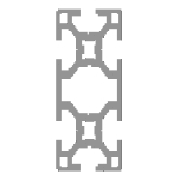
# Autodesk Inventor part: 30-3060
Saved by Autodesk Inventor 2021 (Build 250183000, 183)
## iProperties
Created: 2020-11-08
Part Number: 30-3060
Material: Generic
Document SubType Name: Modeling
Designer: Wes
Manufacturer: 8020
Standards Organization: 8020 Metric
Language: en-US
Size Designation: 30-3060
Categories: <MemberInstance><Categories><Category DisplayName="Structural Shapes" InternalName="089c4875-fa83-4c05-b084-43b9cc11f5ed" Mnemonic="GRDR"><CategoryParameter DisplayName="Mass per Length Unit" InternalName="0bb95a10-148f-4027-a459-38d7b056702a" Mnemonic="shpmass"/><CategoryParameter DisplayName="Section Area" InternalName="1ff91680-64b0-4202-b9a3-7fd3f94bba3b" Mnemonic="secarea"/><CategoryParameter DisplayName="Radius of Gyration (x)" InternalName="25778675-03e9-40c1-b6a8-4a9ed693320d" Mnemonic="gyrradx"/><CategoryParameter DisplayName="Torsional Rigidity Modulus" InternalName="26c1ec35-5026-4c63-ad0a-751cf684a536" Mnemonic="torrigmod"/><CategoryParameter DisplayName="Distance of the Center of Gravity X-X" InternalName="26c9bdb8-9c79-4b4f-a92e-8e197583c9c4" Mnemonic="grcendistX"/><CategoryParameter DisplayName="Legacy Member ID" InternalName="340afe4f-75d7-48d3-ab7d-943f3c3da468" Mnemonic="LegacyMemberID"/><CategoryParameter DisplayName="Base Length" InternalName="42e34263-8f20-4d0e-ad48-bf1385b87c24" Mnemonic="shplen"/><CategoryParameter DisplayName="Moment of Inertia (y)" InternalName="4b9f58ea-bced-460e-81ea-3d29ca5a49e3" Mnemonic="inermomy"/><CategoryParameter DisplayName="Moment of Inertia (x)" InternalName="4cd780bc-73d7-43ac-917a-579e5cbd684d" Mnemonic="inermomx"/><CategoryParameter DisplayName="Custom Base Point" InternalName="4f1d1b73-316d-484b-a3df-9cbabb16eb77" Mnemonic="shpBasePoint"/><CategoryParameter DisplayName="Shape Height" InternalName="50274e7d-5ac0-4796-92cb-c59e54983c67" Mnemonic="shpheig"/><CategoryParameter DisplayName="Section Module (y)" InternalName="59eaa5e9-d227-48dc-b6c1-6920f96e0f95" Mnemonic="secmody"/><CategoryParameter DisplayName="Section Designation" InternalName="5a64d034-428d-49c8-ba32-7619764de20f" Mnemonic="shpdes"/><CategoryParameter DisplayName="Section Module (x)" InternalName="72cfad18-cf51-4ed4-aaa7-c6b224f8419f" Mnemonic="secmodx"/><CategoryParameter DisplayName="Torsional Section Modulus" InternalName="7c55a8dc-8844-49f9-a867-cc677b30ec9a" Mnemonic="torsecmod"/><CategoryParameter DisplayName="Shape Width" InternalName="7c717d54-a18f-4666-b4d4-573cce22c62c" Mnemonic="shpwdth"/><CategoryParameter DisplayName="Second Shape Thickness" InternalName="9251a8e1-85fd-4e47-af99-afdb762317d9" Mnemonic="shpthick2"/><CategoryParameter DisplayName="FG Authored" InternalName="9c666724-f362-4ea7-ac62-f6a007de5c69" Mnemonic="shpFGAuto"/><CategoryParameter DisplayName="Distance of the Center of Gravity Y-Y" InternalName="bcc4fb17-7af4-436a-8f8c-d0aa3b0248c5" Mnemonic="grcendistY"/><CategoryParameter DisplayName="Radius of Gyration (y)" InternalName="bfa18ebe-1636-4dbe-8d42-b263e0b73184" Mnemonic="gyrrady"/><CategoryParameter DisplayName="Shape Thickness" InternalName="d109cf76-8eb4-42fc-9800-4409734adc67" Mnemonic="shpthick"/><CategoryParameter DisplayName="Coefficient of Shear Displacement" InternalName="de4c90c6-aaa8-468f-a335-6737b311b5d3" Mnemonic="shdispc"/><Category DisplayName="Other" InternalName="f02205ff-2390-476f-921c-0b3185f88e84" Mnemonic="OTHSHP"><CategoryParameter DisplayName="Moment of Inertia (y)" InternalName="044c654e-f649-48ac-84cc-650a29ae31ca" Mnemonic="inermomy"/><CategoryParameter DisplayName="Shape Thickness" InternalName="12b1a788-9233-48fd-a933-2df8ff42b15f" Mnemonic="shpthick"/><CategoryParameter DisplayName="Mass per Length Unit" InternalName="2fd289d6-9394-4d2d-97e6-6659d7d4551d" Mnemonic="shpmass"/><CategoryParameter DisplayName="Radius of Gyration (y)" InternalName="743e1dfe-1bba-408b-b985-cf752b207386" Mnemonic="gyrrady"/><CategoryParameter DisplayName="Section Module (y)" InternalName="88b8bff9-a616-4028-93d5-ed4f79680d13" Mnemonic="secmody"/><CategoryParameter DisplayName="Section Area" InternalName="c46ecdf8-b6eb-4db9-8b25-30258930c1e3" Mnemonic="secarea"/><CategoryParameter DisplayName="Section Module (x)" InternalName="cac70804-9d39-43bb-be17-56ea1f39a6c2" Mnemonic="secmodx"/><CategoryParameter DisplayName="Moment of Inertia (x)" InternalName="ec6737bc-264f-43ed-b0bd-f6d410c2718d" Mnemonic="inermomx"/><CategoryParameter DisplayName="Radius of Gyration (x)" InternalName="ee72c61e-565e-4fd6-b448-66e1e1abcb7e" Mnemonic="gyrradx"/><Category DisplayName="8020" InternalName="79851eee-1260-43d5-80eb-d25638456875" Mnemonic="8020"/></Category></Category><Category DisplayName="DataType" InternalName="23b78d0f-2648-40c6-8793-ca6db495c9e8" Mnemonic="DATATYPE"><CategoryParameter DisplayName="DisplayName" InternalName="05415f3d-3907-474b-a020-eb9d644f4cf3" Mnemonic="DISPLAYNAME"/><CategoryParameter DisplayName="Standard" InternalName="0c0a119c-1e12-4c84-803f-101930972f5e" Mnemonic="STANDARD"/><CategoryParameter DisplayName="Description" InternalName="13903e3d-64b1-4950-80da-f627842ea37f" Mnemonic="DESCRIPTION"/><CategoryParameter DisplayName="Designation" InternalName="2675968c-4ce5-49e0-a4f5-552d29089031" Mnemonic="DESIGNATION"/><CategoryParameter DisplayName="Default Row" InternalName="2af9ec52-faaa-4026-b378-f9fa4afca842" Mnemonic="DEFAULTROW"/><CategoryParameter DisplayName="Folder Name" InternalName="3f06958e-8713-4116-9be7-ed6184ecc97b" Mnemonic="FOLDERNAME"/><CategoryParameter DisplayName="Revision Guid" InternalName="45a75005-10b1-4dfc-8d6d-dfe629f0b93c" Mnemonic="REVISIONGUID"/><CategoryParameter DisplayName="FileName" InternalName="8b46a4cc-9585-4fed-90c3-899f57e09a73" Mnemonic="FILENAME"/><CategoryParameter DisplayName="StdsOrg" InternalName="8f5914e1-4693-403f-8ab5-d37768198c9d" Mnemonic="STDSORG"/><CategoryParameter DisplayName="Family Version" InternalName="914462f6-6e19-4b14-ba84-155b9680b1d0" Mnemonic="FAMILYREVISION"/><CategoryParameter DisplayName="Standard Revision" InternalName="91d5a463-65c2-4fde-b823-3b7fea5e8e17" Mnemonic="STANDARDREVISION"/><CategoryParameter DisplayName="Member Revision" InternalName="a65d44b9-392f-4f4f-857b-e4b3d54996fe" Mnemonic="MEMBERREVISION"/><CategoryParameter DisplayName="ClipFormat" InternalName="bc51e27b-3422-4e78-93ef-cec197ddf230" Mnemonic="CLIPFORMAT"/><CategoryParameter DisplayName="Manufacturer" InternalName="cd6c7a72-a28a-4e50-99a9-2c7f4e13e5ad" Mnemonic="MANUFACTURER"/><CategoryParameter DisplayName="InternalName" InternalName="cf1d0246-76d9-4b4a-8305-fa0409afb5c1" Mnemonic="INTERNALNAME"/><CategoryParameter DisplayName="IsMetric" InternalName="e2385c5b-1ea4-4823-96a8-8de651266ec3" Mnemonic="ISMETRIC"/><Category DisplayName="Part" InternalName="c0e0b642-3bcb-4cc8-9e80-f96d35c4afa4" Mnemonic="PART"><CategoryParameter DisplayName="Part Number" InternalName="016b6077-bfbe-49bd-92c9-d8d59c39c941" Mnemonic="PARTNUMBER"/><CategoryParameter DisplayName="Stock Number" InternalName="4dba7c1c-e26c-444e-836c-b08b433409a8" Mnemonic="STOCKNUMBER"/><CategoryParameter DisplayName="Material Key" InternalName="5c9a8adb-dd2b-4535-b97f-0a94a95fe41f" Mnemonic="MATERIALKEY"/><CategoryParameter DisplayName="Material" InternalName="818a152a-d3c3-49ca-80ee-df7d91421b8e" Mnemonic="MATERIAL"/></Category></Category></Categories><FamilyTemplate Id="30-3060"><FamilyTemplateParameters><FamilyTemplateParameter ObjectType="kModelParameterObject" ValueType="xs:double" Id="12" ObjectReferenceKey="Length"/><FamilyTemplateParameter ObjectType="kPartComponentDefinitionObject" ValueType="xs:string" Id="23" SubObjectId="Material"/><FamilyTemplateParameter ObjectType="kPropertyObject" ValueType="xs:string" Id="26" ObjectReferenceKey="{32853F0F-3444-11d1-9E93-0060B03C1CA6}" SubObjectId="5"/><FamilyTemplateParameter ObjectType="kPropertyObject" ValueType="xs:string" Id="27" ObjectReferenceKey="{32853F0F-3444-11d1-9E93-0060B03C1CA6}" SubObjectId="52"/></FamilyTemplateParameters></FamilyTemplate><CategoryParameterMap><ParamToTemplateMap><ParamToTemplate CategoryParameter="//CategoryParameter[@InternalName='cf1d0246-76d9-4b4a-8305-fa0409afb5c1']" ConstantValue="ebd6c703-6585-4f80-969f-cab21f52a046"/><ParamToTemplate CategoryParameter="//CategoryParameter[@InternalName='45a75005-10b1-4dfc-8d6d-dfe629f0b93c']" ConstantValue="7500c355-f6d2-45da-9c20-dd8006f12ffd"/><ParamToTemplate CategoryParameter="//CategoryParameter[@InternalName='3f06958e-8713-4116-9be7-ed6184ecc97b']" ConstantValue="30-3060"/><ParamToTemplate CategoryParameter="//CategoryParameter[@InternalName='8f5914e1-4693-403f-8ab5-d37768198c9d']" ConstantValue="8020 Metric"/><ParamToTemplate CategoryParameter="//CategoryParameter[@InternalName='0c0a119c-1e12-4c84-803f-101930972f5e']" TemplateParameter="18"/><ParamToTemplate CategoryParameter="//CategoryParameter[@InternalName='91d5a463-65c2-4fde-b823-3b7fea5e8e17']" TemplateParameter="19"/><ParamToTemplate CategoryParameter="//CategoryParameter[@InternalName='cd6c7a72-a28a-4e50-99a9-2c7f4e13e5ad']" ConstantValue="8020"/><ParamToTemplate CategoryParameter="//CategoryParameter[@InternalName='13903e3d-64b1-4950-80da-f627842ea37f']" TemplateParameter="22"/><ParamToTemplate CategoryParameter="//CategoryParameter[@InternalName='05415f3d-3907-474b-a020-eb9d644f4cf3']" ConstantValue="30-3060"/><ParamToTemplate CategoryParameter="//CategoryParameter[@InternalName='914462f6-6e19-4b14-ba84-155b9680b1d0']" ConstantValue="11"/><ParamToTemplate CategoryParameter="//CategoryParameter[@InternalName='bc51e27b-3422-4e78-93ef-cec197ddf230']" ConstantValue="CF_INVENTOR.STDPARTS"/><ParamToTemplate CategoryParameter="//CategoryParameter[@InternalName='e2385c5b-1ea4-4823-96a8-8de651266ec3']" ConstantValue="false"/><ParamToTemplate CategoryParameter="//CategoryParameter[@InternalName='2af9ec52-faaa-4026-b378-f9fa4afca842']" ConstantValue="1"/><ParamToTemplate CategoryParameter="//CategoryParameter[@InternalName='4f1d1b73-316d-484b-a3df-9cbabb16eb77']" ConstantValue="1"/><ParamToTemplate CategoryParameter="//CategoryParameter[@InternalName='9c666724-f362-4ea7-ac62-f6a007de5c69']" ConstantValue="1"/><ParamToTemplate CategoryParameter="//CategoryParameter[@InternalName='8b46a4cc-9585-4fed-90c3-899f57e09a73']" ConstantValue="30-3060"/><ParamToTemplate CategoryParameter="//CategoryParameter[@InternalName='a65d44b9-392f-4f4f-857b-e4b3d54996fe']" ConstantValue="3621f859-3cd7-4c8d-9d7e-184ee6a29b8c"/><ParamToTemplate CategoryParameter="//CategoryParameter[@InternalName='a65d44b9-392f-4f4f-857b-e4b3d54996fe']" ConstantValue="3621f859-3cd7-4c8d-9d7e-184ee6a29b8c"/><ParamToTemplate CategoryParameter="//CategoryParameter[@InternalName='2675968c-4ce5-49e0-a4f5-552d29089031']" TemplateParameter="27"/><ParamToTemplate CategoryParameter="//CategoryParameter[@InternalName='42e34263-8f20-4d0e-ad48-bf1385b87c24']" TemplateParameter="12"/><ParamToTemplate CategoryParameter="//CategoryParameter[@InternalName='818a152a-d3c3-49ca-80ee-df7d91421b8e']" TemplateParameter="23"/><ParamToTemplate CategoryParameter="//CategoryParameter[@InternalName='016b6077-bfbe-49bd-92c9-d8d59c39c941']" TemplateParameter="26"/></ParamToTemplateMap></CategoryParameterMap></MemberInstance>
Density: 1 g/cm^3
Appearance: Default
_CCFamilyDisplayName: 30-3060
_FrameMemberDoc: Frame Member File
_Version: 15.0.0
_GetPNFromCC: 1
IsCustomPart: 1
G_W: 1.181 in
G_H: 2.362 in
+1E485C6B-74E4-4670-9E51-72C930FDFDFE+CUTDETAIL2: Cut Angle 90.00 deg
G_L: 30.472 in
+ECDC0DF4-1E61-4BE6-A4E6-B4BFEEAFBB01+CUTDETAIL1: Cut Angle 90.00 deg
Author: Wes
Autodesk Inventor part; units mm, degrees
sketch "30-3060" plane through (0, 0, 0) normal (0, 0, 1) x (1, 0, 0)
  arc A0 (20.0319, 67.4331) -> (20.4119, 67.0531) centre (20.4119, 67.4331) ccw
  line L0 (20.4119, 67.0531) -> (23.8509, 67.0531)
  arc A1 (23.8509, 67.0531) -> (24.2319, 67.4341) centre (23.8509, 67.4341) ccw
  line L1 (24.2319, 67.4341) -> (24.2319, 70.2531)
  arc A2 (24.2319, 70.2531) -> (23.2319, 71.2531) centre (23.2319, 70.2531) ccw
  line L2 (23.2319, 71.2531) -> (20.4129, 71.2531)
  arc A3 (20.4129, 71.2531) -> (20.0319, 70.8721) centre (20.4129, 70.8721) ccw
  line L3 (20.0319, 70.8721) -> (20.0319, 67.4331)
  arc A4 (14.357, 59.8716) -> (12.8504, 61.3782) centre (13.5193, 60.5405) ccw
  line L4 (12.8504, 61.3782) -> (11.8713, 60.5964)
  arc A5 (11.8713, 60.5964) -> (9.1833, 60.5923) centre (10.5319, 57.5531) ccw
  line L5 (9.1833, 60.5923) -> (8.2041, 61.3741)
  arc A6 (8.2041, 61.3741) -> (6.6976, 59.8675) centre (7.5353, 60.5364) ccw
  line L6 (6.6976, 59.8675) -> (7.4842, 58.8824)
  arc A7 (7.4842, 58.8824) -> (7.4886, 56.2137) centre (10.5319, 57.5531) ccw
  line L7 (7.4886, 56.2137) -> (6.7068, 55.2346)
  arc A8 (6.7068, 55.2346) -> (8.2134, 53.728) centre (7.5445, 54.5657) ccw
  line L8 (8.2134, 53.728) -> (9.1925, 54.5098)
  arc A9 (9.1925, 54.5098) -> (11.8713, 54.5098) centre (10.5319, 57.5531) ccw
  line L9 (11.8713, 54.5098) -> (12.8504, 53.728)
  arc A10 (12.8504, 53.728) -> (14.357, 55.2346) centre (13.5193, 54.5657) ccw
  line L10 (14.357, 55.2346) -> (13.5752, 56.2137)
  arc A11 (13.5752, 56.2137) -> (13.5752, 58.8925) centre (10.5319, 57.5531) ccw
  line L11 (13.5752, 58.8925) -> (14.357, 59.8716)
  arc A12 (14.357, 29.8717) -> (12.8504, 31.3783) centre (13.5193, 30.5406) ccw
  line L12 (12.8504, 31.3783) -> (11.8713, 30.5965)
  arc A13 (11.8713, 30.5965) -> (9.1833, 30.5924) centre (10.5319, 27.5532) ccw
  line L13 (9.1833, 30.5924) -> (8.2041, 31.3742)
  arc A14 (8.2041, 31.3742) -> (6.6976, 29.8676) centre (7.5353, 30.5365) ccw
  line L14 (6.6976, 29.8676) -> (7.4842, 28.8824)
  arc A15 (7.4842, 28.8824) -> (7.4886, 26.2138) centre (10.5319, 27.5532) ccw
  line L15 (7.4886, 26.2138) -> (6.7068, 25.2347)
  arc A16 (6.7068, 25.2347) -> (8.2134, 23.7281) centre (7.5445, 24.5658) ccw
  line L16 (8.2134, 23.7281) -> (9.1925, 24.5099)
  arc A17 (9.1925, 24.5099) -> (11.8713, 24.5099) centre (10.5319, 27.5532) ccw
  line L17 (11.8713, 24.5099) -> (12.8504, 23.7281)
  arc A18 (12.8504, 23.7281) -> (14.357, 25.2347) centre (13.5193, 24.5658) ccw
  line L18 (14.357, 25.2347) -> (13.5752, 26.2138)
  arc A19 (13.5752, 26.2138) -> (13.5752, 28.8926) centre (10.5319, 27.5532) ccw
  line L19 (13.5752, 28.8926) -> (14.357, 29.8717)
  arc A20 (23.2319, 13.8532) -> (24.2319, 14.8532) centre (23.2319, 14.8532) ccw
  line L20 (24.2319, 14.8532) -> (24.2319, 17.6722)
  arc A21 (24.2319, 17.6722) -> (23.8509, 18.0532) centre (23.8509, 17.6722) ccw
  line L21 (23.8509, 18.0532) -> (20.4119, 18.0532)
  arc A22 (20.4119, 18.0532) -> (20.0319, 17.6732) centre (20.4119, 17.6732) ccw
  line L22 (20.0319, 17.6732) -> (20.0319, 14.2342)
  arc A23 (20.0319, 14.2342) -> (20.4129, 13.8532) centre (20.4129, 14.2342) ccw
  line L23 (20.4129, 13.8532) -> (23.2319, 13.8532)
  line L24 (-2.2106, 49.8206) -> (-2.2106, 52.9906)
  arc A24 (-2.2106, 49.8206) -> (-1.7109, 49.3031) centre (-1.7109, 49.8031) ccw
  line L25 (0.2717, 49.3031) -> (-1.7109, 49.3031)
  arc A25 (0.2717, 49.3031) -> (0.6252, 49.4496) centre (0.2717, 49.8031) ccw
  line L26 (4.5508, 53.3751) -> (0.6252, 49.4496)
  arc A26 (4.5508, 53.3751) -> (4.6972, 53.7287) centre (4.1972, 53.7287) ccw
  line L27 (4.6972, 56.6031) -> (4.6972, 53.7287)
  line L28 (5.2072, 57.5531) -> (4.6972, 56.6031)
  line L29 (4.6972, 58.5031) -> (5.2072, 57.5531)
  line L30 (4.6972, 61.3776) -> (4.6972, 58.5031)
  arc A27 (4.6972, 61.3776) -> (4.5508, 61.7311) centre (4.1972, 61.3776) ccw
  line L31 (0.6252, 65.6567) -> (4.5508, 61.7311)
  arc A28 (0.6252, 65.6567) -> (0.2717, 65.8031) centre (0.2717, 65.3031) ccw
  line L32 (-1.7109, 65.8031) -> (0.2717, 65.8031)
  arc A29 (-1.7109, 65.8031) -> (-2.2106, 65.2857) centre (-1.7109, 65.3031) ccw
  line L33 (-2.2106, 61.9906) -> (-2.2106, 65.2857)
  arc A30 (-2.7106, 61.4906) -> (-2.2106, 61.9906) centre (-2.7106, 61.9906) ccw
  line L34 (-3.9681, 61.4906) -> (-2.7106, 61.4906)
  arc A31 (-4.4681, 61.9906) -> (-3.9681, 61.4906) centre (-3.9681, 61.9906) ccw
  line L35 (-4.4681, 70.5531) -> (-4.4681, 61.9906)
  arc A32 (-2.4681, 72.5531) -> (-4.4681, 70.5531) centre (-2.4681, 70.5531) ccw
  line L36 (5.9694, 72.5531) -> (-2.4681, 72.5531)
  arc A33 (6.4694, 72.0531) -> (5.9694, 72.5531) centre (5.9694, 72.0531) ccw
  line L37 (6.4694, 70.7956) -> (6.4694, 72.0531)
  arc A34 (5.9694, 70.2956) -> (6.4694, 70.7956) centre (5.9694, 70.7956) ccw
  line L38 (2.7994, 70.2956) -> (5.9694, 70.2956)
  arc A35 (2.7994, 70.2956) -> (2.2819, 69.7959) centre (2.7819, 69.7959) ccw
  line L39 (2.2819, 67.8133) -> (2.2819, 69.7959)
  arc A36 (2.2819, 67.8133) -> (2.4284, 67.4598) centre (2.7819, 67.8133) ccw
  line L40 (6.3539, 63.5342) -> (2.4284, 67.4598)
  arc A37 (6.3539, 63.5342) -> (6.7074, 63.3878) centre (6.7074, 63.8878) ccw
  line L41 (9.5194, 63.3878) -> (6.7074, 63.3878)
  line L42 (10.4694, 62.8778) -> (9.5194, 63.3878)
  line L43 (11.4194, 63.3878) -> (10.4694, 62.8778)
  line L44 (14.3564, 63.3878) -> (11.4194, 63.3878)
  arc A38 (14.3564, 63.3878) -> (14.7099, 63.5342) centre (14.3564, 63.8878) ccw
  line L45 (18.6354, 67.4598) -> (14.7099, 63.5342)
  arc A39 (18.6354, 67.4598) -> (18.7819, 67.8133) centre (18.2819, 67.8133) ccw
  line L46 (18.7819, 69.7959) -> (18.7819, 67.8133)
  arc A40 (18.7819, 69.7959) -> (18.2644, 70.2956) centre (18.2819, 69.7959) ccw
  line L47 (14.9694, 70.2956) -> (18.2644, 70.2956)
  arc A41 (14.4694, 70.7956) -> (14.9694, 70.2956) centre (14.9694, 70.7956) ccw
  line L48 (14.4694, 72.0531) -> (14.4694, 70.7956)
  arc A42 (14.9694, 72.5531) -> (14.4694, 72.0531) centre (14.9694, 72.0531) ccw
  line L49 (23.5319, 72.5531) -> (14.9694, 72.5531)
  arc A43 (25.5319, 70.5531) -> (23.5319, 72.5531) centre (23.5319, 70.5531) ccw
  line L50 (25.5319, 62.1156) -> (25.5319, 70.5531)
  arc A44 (25.0319, 61.6156) -> (25.5319, 62.1156) centre (25.0319, 62.1156) ccw
  line L51 (23.7744, 61.6156) -> (25.0319, 61.6156)
  arc A45 (23.2744, 62.1156) -> (23.7744, 61.6156) centre (23.7744, 62.1156) ccw
  line L52 (23.2744, 65.2857) -> (23.2744, 62.1156)
  arc A46 (23.2744, 65.2857) -> (22.7747, 65.8031) centre (22.7747, 65.3031) ccw
  line L53 (20.7921, 65.8031) -> (22.7747, 65.8031)
  arc A47 (20.7921, 65.8031) -> (20.4386, 65.6567) centre (20.7921, 65.3031) ccw
  line L54 (16.513, 61.7311) -> (20.4386, 65.6567)
  arc A48 (16.513, 61.7311) -> (16.3666, 61.3776) centre (16.8666, 61.3776) ccw
  line L55 (16.3666, 58.5031) -> (16.3666, 61.3776)
  line L56 (15.8566, 57.5531) -> (16.3666, 58.5031)
  line L57 (16.3666, 56.6031) -> (15.8566, 57.5531)
  line L58 (16.3666, 53.7287) -> (16.3666, 56.6031)
  arc A49 (16.3666, 53.7287) -> (16.513, 53.3751) centre (16.8666, 53.7287) ccw
  line L59 (20.4386, 49.4496) -> (16.513, 53.3751)
  arc A50 (20.4386, 49.4496) -> (20.7921, 49.3031) centre (20.7921, 49.8031) ccw
  line L60 (22.7747, 49.3031) -> (20.7921, 49.3031)
  arc A51 (22.7747, 49.3031) -> (23.2744, 49.8206) centre (22.7747, 49.8031) ccw
  line L61 (23.2744, 53.1156) -> (23.2744, 49.8206)
  arc A52 (23.7744, 53.6156) -> (23.2744, 53.1156) centre (23.7744, 53.1156) ccw
  line L62 (25.0319, 53.6156) -> (23.7744, 53.6156)
  arc A53 (25.5319, 53.1156) -> (25.0319, 53.6156) centre (25.0319, 53.1156) ccw
  line L63 (25.5319, 31.9907) -> (25.5319, 53.1156)
  arc A54 (25.0319, 31.4907) -> (25.5319, 31.9907) centre (25.0319, 31.9907) ccw
  line L64 (23.7744, 31.4907) -> (25.0319, 31.4907)
  arc A55 (23.2744, 31.9907) -> (23.7744, 31.4907) centre (23.7744, 31.9907) ccw
  line L65 (23.2744, 35.2857) -> (23.2744, 31.9907)
  arc A56 (23.2744, 35.2857) -> (22.7747, 35.8032) centre (22.7747, 35.3032) ccw
  line L66 (20.7921, 35.8032) -> (22.7747, 35.8032)
  arc A57 (20.7921, 35.8032) -> (20.4386, 35.6567) centre (20.7921, 35.3032) ccw
  line L67 (16.513, 31.7312) -> (20.4386, 35.6567)
  arc A58 (16.513, 31.7312) -> (16.3666, 31.3776) centre (16.8666, 31.3776) ccw
  line L68 (16.3666, 28.5032) -> (16.3666, 31.3776)
  line L69 (15.8566, 27.5532) -> (16.3666, 28.5032)
  line L70 (16.3666, 26.6032) -> (15.8566, 27.5532)
  line L71 (16.3666, 23.7287) -> (16.3666, 26.6032)
  arc A59 (16.3666, 23.7287) -> (16.513, 23.3752) centre (16.8666, 23.7287) ccw
  line L72 (20.4386, 19.4496) -> (16.513, 23.3752)
  arc A60 (20.4386, 19.4496) -> (20.7921, 19.3032) centre (20.7921, 19.8032) ccw
  line L73 (22.7747, 19.3032) -> (20.7921, 19.3032)
  arc A61 (22.7747, 19.3032) -> (23.2744, 19.8206) centre (22.7747, 19.8032) ccw
  line L74 (23.2744, 22.9907) -> (23.2744, 19.8206)
  arc A62 (23.7744, 23.4907) -> (23.2744, 22.9907) centre (23.7744, 22.9907) ccw
  line L75 (25.0319, 23.4907) -> (23.7744, 23.4907)
  arc A63 (25.5319, 22.9907) -> (25.0319, 23.4907) centre (25.0319, 22.9907) ccw
  line L76 (25.5319, 14.5532) -> (25.5319, 22.9907)
  arc A64 (23.5319, 12.5532) -> (25.5319, 14.5532) centre (23.5319, 14.5532) ccw
  line L77 (14.9694, 12.5532) -> (23.5319, 12.5532)
  arc A65 (14.4694, 13.0532) -> (14.9694, 12.5532) centre (14.9694, 13.0532) ccw
  line L78 (14.4694, 14.3107) -> (14.4694, 13.0532)
  arc A66 (14.9694, 14.8107) -> (14.4694, 14.3107) centre (14.9694, 14.3107) ccw
  line L79 (18.2644, 14.8107) -> (14.9694, 14.8107)
  arc A67 (18.2644, 14.8107) -> (18.7819, 15.3104) centre (18.2819, 15.3104) ccw
  line L80 (18.7819, 17.293) -> (18.7819, 15.3104)
  arc A68 (18.7819, 17.293) -> (18.6354, 17.6465) centre (18.2819, 17.293) ccw
  line L81 (14.7099, 21.572) -> (18.6354, 17.6465)
  arc A69 (14.7099, 21.572) -> (14.3564, 21.7185) centre (14.3564, 21.2185) ccw
  line L82 (11.4194, 21.7185) -> (14.3564, 21.7185)
  line L83 (10.4694, 22.2285) -> (11.4194, 21.7185)
  line L84 (9.5194, 21.7185) -> (10.4694, 22.2285)
  line L85 (6.7074, 21.7185) -> (9.5194, 21.7185)
  arc A70 (6.7074, 21.7185) -> (6.3539, 21.572) centre (6.7074, 21.2185) ccw
  line L86 (2.4284, 17.6465) -> (6.3539, 21.572)
  arc A71 (2.4284, 17.6465) -> (2.2819, 17.293) centre (2.7819, 17.293) ccw
  line L87 (2.2819, 15.3104) -> (2.2819, 17.293)
  arc A72 (2.2819, 15.3104) -> (2.7994, 14.8107) centre (2.7819, 15.3104) ccw
  line L88 (5.9694, 14.8107) -> (2.7994, 14.8107)
  arc A73 (6.4694, 14.3107) -> (5.9694, 14.8107) centre (5.9694, 14.3107) ccw
  line L89 (6.4694, 13.0532) -> (6.4694, 14.3107)
  arc A74 (5.9694, 12.5532) -> (6.4694, 13.0532) centre (5.9694, 13.0532) ccw
  line L90 (-2.4681, 12.5532) -> (5.9694, 12.5532)
  arc A75 (-4.4681, 14.5532) -> (-2.4681, 12.5532) centre (-2.4681, 14.5532) ccw
  line L91 (-4.4681, 23.1157) -> (-4.4681, 14.5532)
  arc A76 (-3.9681, 23.6157) -> (-4.4681, 23.1157) centre (-3.9681, 23.1157) ccw
  line L92 (-2.7106, 23.6157) -> (-3.9681, 23.6157)
  arc A77 (-2.2106, 23.1157) -> (-2.7106, 23.6157) centre (-2.7106, 23.1157) ccw
  line L93 (-2.2106, 19.8206) -> (-2.2106, 23.1157)
  arc A78 (-2.2106, 19.8206) -> (-1.7109, 19.3032) centre (-1.7109, 19.8032) ccw
  line L94 (0.2717, 19.3032) -> (-1.7109, 19.3032)
  arc A79 (0.2717, 19.3032) -> (0.6252, 19.4496) centre (0.2717, 19.8032) ccw
  line L95 (4.5508, 23.3752) -> (0.6252, 19.4496)
  arc A80 (4.5508, 23.3752) -> (4.6972, 23.7287) centre (4.1972, 23.7287) ccw
  line L96 (4.6972, 26.6032) -> (4.6972, 23.7287)
  line L97 (5.2072, 27.5532) -> (4.6972, 26.6032)
  line L98 (4.6972, 28.5032) -> (5.2072, 27.5532)
  line L99 (4.6972, 31.3776) -> (4.6972, 28.5032)
  arc A81 (4.6972, 31.3776) -> (4.5508, 31.7312) centre (4.1972, 31.3776) ccw
  line L100 (0.6252, 35.6567) -> (4.5508, 31.7312)
  arc A82 (0.6252, 35.6567) -> (0.2717, 35.8032) centre (0.2717, 35.3032) ccw
  line L101 (-1.7109, 35.8032) -> (0.2717, 35.8032)
  arc A83 (-1.7109, 35.8032) -> (-2.2106, 35.2857) centre (-1.7109, 35.3032) ccw
  line L102 (-2.2106, 32.1157) -> (-2.2106, 35.2857)
  arc A84 (-2.7106, 31.6157) -> (-2.2106, 32.1157) centre (-2.7106, 32.1157) ccw
  line L103 (-3.9681, 31.6157) -> (-2.7106, 31.6157)
  arc A85 (-4.4681, 32.1157) -> (-3.9681, 31.6157) centre (-3.9681, 32.1157) ccw
  line L104 (-4.4681, 52.9906) -> (-4.4681, 32.1157)
  arc A86 (-3.9681, 53.4906) -> (-4.4681, 52.9906) centre (-3.9681, 52.9906) ccw
  line L105 (-2.7106, 53.4906) -> (-3.9681, 53.4906)
  arc A87 (-2.2106, 52.9906) -> (-2.7106, 53.4906) centre (-2.7106, 52.9906) ccw
  arc A88 (1.0319, 17.6732) -> (0.6519, 18.0532) centre (0.6519, 17.6732) ccw
  line L106 (0.6519, 18.0532) -> (-2.7871, 18.0532)
  arc A89 (-2.7871, 18.0532) -> (-3.1681, 17.6722) centre (-2.7871, 17.6722) ccw
  line L107 (-3.1681, 17.6722) -> (-3.1681, 14.8532)
  arc A90 (-3.1681, 14.8532) -> (-2.1681, 13.8532) centre (-2.1681, 14.8532) ccw
  line L108 (-2.1681, 13.8532) -> (0.6509, 13.8532)
  arc A91 (0.6509, 13.8532) -> (1.0319, 14.2342) centre (0.6509, 14.2342) ccw
  line L109 (1.0319, 14.2342) -> (1.0319, 17.6732)
  arc A92 (23.3319, 46.6031) -> (22.8319, 47.1031) centre (22.8319, 46.6031) ccw
  line L110 (22.8319, 47.1031) -> (19.8001, 47.1031)
  arc A93 (18.7394, 47.5425) -> (19.8001, 47.1031) centre (19.8001, 48.6031) ccw
  line L111 (18.7394, 47.5425) -> (14.7099, 51.572)
  arc A94 (14.7099, 51.572) -> (14.3564, 51.7184) centre (14.3564, 51.2184) ccw
  line L112 (14.3564, 51.7184) -> (11.4194, 51.7184)
  line L113 (11.4194, 51.7184) -> (10.4694, 52.2284)
  line L114 (10.4694, 52.2284) -> (9.5194, 51.7184)
  line L115 (9.5194, 51.7184) -> (6.7074, 51.7184)
  arc A95 (6.7074, 51.7184) -> (6.3539, 51.572) centre (6.7074, 51.2184) ccw
  line L116 (6.3539, 51.572) -> (2.3244, 47.5425)
  arc A96 (1.2637, 47.1031) -> (2.3244, 47.5425) centre (1.2637, 48.6031) ccw
  line L117 (1.2637, 47.1031) -> (-1.7681, 47.1031)
  arc A97 (-1.7681, 47.1031) -> (-2.2681, 46.6031) centre (-1.7681, 46.6031) ccw
  line L118 (-2.2681, 46.6031) -> (-2.2681, 38.5032)
  arc A98 (-2.2681, 38.5032) -> (-1.7681, 38.0032) centre (-1.7681, 38.5032) ccw
  line L119 (-1.7681, 38.0032) -> (1.2637, 38.0032)
  arc A99 (2.3244, 37.5638) -> (1.2637, 38.0032) centre (1.2637, 36.5032) ccw
  line L120 (2.3244, 37.5638) -> (6.3539, 33.5343)
  arc A100 (6.3539, 33.5343) -> (6.7074, 33.3879) centre (6.7074, 33.8879) ccw
  line L121 (6.7074, 33.3879) -> (9.5194, 33.3879)
  line L122 (9.5194, 33.3879) -> (10.4694, 32.8779)
  line L123 (10.4694, 32.8779) -> (11.4194, 33.3879)
  line L124 (11.4194, 33.3879) -> (14.3564, 33.3879)
  arc A101 (14.3564, 33.3879) -> (14.7099, 33.5343) centre (14.3564, 33.8879) ccw
  line L125 (14.7099, 33.5343) -> (18.7394, 37.5638)
  arc A102 (19.8001, 38.0032) -> (18.7394, 37.5638) centre (19.8001, 36.5032) ccw
  line L126 (19.8001, 38.0032) -> (22.8319, 38.0032)
  arc A103 (22.8319, 38.0032) -> (23.3319, 38.5032) centre (22.8319, 38.5032) ccw
  line L127 (23.3319, 38.5032) -> (23.3319, 46.6031)
  arc A104 (0.6519, 67.0531) -> (1.0319, 67.4331) centre (0.6519, 67.4331) ccw
  line L128 (1.0319, 67.4331) -> (1.0319, 70.8721)
  arc A105 (1.0319, 70.8721) -> (0.6509, 71.2531) centre (0.6509, 70.8721) ccw
  line L129 (0.6509, 71.2531) -> (-2.1681, 71.2531)
  arc A106 (-2.1681, 71.2531) -> (-3.1681, 70.2531) centre (-2.1681, 70.2531) ccw
  line L130 (-3.1681, 70.2531) -> (-3.1681, 67.4341)
  arc A107 (-3.1681, 67.4341) -> (-2.7871, 67.0531) centre (-2.7871, 67.4341) ccw
  line L131 (-2.7871, 67.0531) -> (0.6519, 67.0531)
ref_plane "Start Plane" through (0, 0, 29.9999) normal (0, 0, 1) x (1, 0, 0)
ref_plane "End Plane" through (0, 0, 804.0001) normal (0, 0, 1) x (1, 0, 0)
sketch "Sketch" plane through (0, 0, 0) normal (0, 0, 1) x (1, 0, 0)
  arc A0 (9.5, 39.8799) -> (9.88, 39.4999) centre (9.88, 39.8799) ccw
  line L0 (9.88, 39.4999) -> (13.319, 39.4999)
  arc A1 (13.319, 39.4999) -> (13.7, 39.8809) centre (13.319, 39.8809) ccw
  line L1 (13.7, 39.8809) -> (13.7, 42.6999)
  arc A2 (13.7, 42.6999) -> (12.7, 43.6999) centre (12.7, 42.6999) ccw
  line L2 (12.7, 43.6999) -> (9.881, 43.6999)
  arc A3 (9.881, 43.6999) -> (9.5, 43.3189) centre (9.881, 43.3189) ccw
  line L3 (9.5, 43.3189) -> (9.5, 39.8799)
  arc A4 (3.8251, 32.3184) -> (2.3185, 33.825) centre (2.9874, 32.9873) ccw
  line L4 (2.3185, 33.825) -> (1.3394, 33.0432)
  arc A5 (1.3394, 33.0432) -> (-1.3486, 33.0391) centre (0, 29.9999) ccw
  line L5 (-1.3486, 33.0391) -> (-2.3278, 33.8209)
  arc A6 (-2.3278, 33.8209) -> (-3.8343, 32.3143) centre (-2.9966, 32.9832) ccw
  line L6 (-3.8343, 32.3143) -> (-3.0477, 31.3292)
  arc A7 (-3.0477, 31.3292) -> (-3.0433, 28.6606) centre (0, 29.9999) ccw
  line L7 (-3.0433, 28.6606) -> (-3.8251, 27.6814)
  arc A8 (-3.8251, 27.6814) -> (-2.3185, 26.1749) centre (-2.9874, 27.0126) ccw
  line L8 (-2.3185, 26.1749) -> (-1.3394, 26.9566)
  arc A9 (-1.3394, 26.9566) -> (1.3394, 26.9566) centre (0, 29.9999) ccw
  line L9 (1.3394, 26.9566) -> (2.3185, 26.1749)
  arc A10 (2.3185, 26.1749) -> (3.8251, 27.6814) centre (2.9874, 27.0126) ccw
  line L10 (3.8251, 27.6814) -> (3.0433, 28.6606)
  arc A11 (3.0433, 28.6606) -> (3.0433, 31.3393) centre (0, 29.9999) ccw
  line L11 (3.0433, 31.3393) -> (3.8251, 32.3184)
  arc A12 (3.8251, 2.3185) -> (2.3185, 3.8251) centre (2.9874, 2.9874) ccw
  line L12 (2.3185, 3.8251) -> (1.3394, 3.0433)
  arc A13 (1.3394, 3.0433) -> (-1.3486, 3.0392) centre (0, 0) ccw
  line L13 (-1.3486, 3.0392) -> (-2.3278, 3.821)
  arc A14 (-2.3278, 3.821) -> (-3.8343, 2.3144) centre (-2.9966, 2.9833) ccw
  line L14 (-3.8343, 2.3144) -> (-3.0477, 1.3292)
  arc A15 (-3.0477, 1.3292) -> (-3.0433, -1.3394) centre (0, 0) ccw
  line L15 (-3.0433, -1.3394) -> (-3.8251, -2.3185)
  arc A16 (-3.8251, -2.3185) -> (-2.3185, -3.8251) centre (-2.9874, -2.9874) ccw
  line L16 (-2.3185, -3.8251) -> (-1.3394, -3.0433)
  arc A17 (-1.3394, -3.0433) -> (1.3394, -3.0433) centre (0, 0) ccw
  line L17 (1.3394, -3.0433) -> (2.3185, -3.8251)
  arc A18 (2.3185, -3.8251) -> (3.8251, -2.3185) centre (2.9874, -2.9874) ccw
  line L18 (3.8251, -2.3185) -> (3.0433, -1.3394)
  arc A19 (3.0433, -1.3394) -> (3.0433, 1.3394) centre (0, 0) ccw
  line L19 (3.0433, 1.3394) -> (3.8251, 2.3185)
  arc A20 (12.7, -13.7) -> (13.7, -12.7) centre (12.7, -12.7) ccw
  line L20 (13.7, -12.7) -> (13.7, -9.881)
  arc A21 (13.7, -9.881) -> (13.319, -9.5) centre (13.319, -9.881) ccw
  line L21 (13.319, -9.5) -> (9.88, -9.5)
  arc A22 (9.88, -9.5) -> (9.5, -9.88) centre (9.88, -9.88) ccw
  line L22 (9.5, -9.88) -> (9.5, -13.319)
  arc A23 (9.5, -13.319) -> (9.881, -13.7) centre (9.881, -13.319) ccw
  line L23 (9.881, -13.7) -> (12.7, -13.7)
  line L24 (-12.7425, 22.2674) -> (-12.7425, 25.4374)
  arc A24 (-12.7425, 22.2674) -> (-12.2428, 21.75) centre (-12.2428, 22.25) ccw
  line L25 (-10.2602, 21.75) -> (-12.2428, 21.75)
  arc A25 (-10.2602, 21.75) -> (-9.9067, 21.8964) centre (-10.2602, 22.25) ccw
  line L26 (-5.9811, 25.8219) -> (-9.9067, 21.8964)
  arc A26 (-5.9811, 25.8219) -> (-5.8347, 26.1755) centre (-6.3347, 26.1755) ccw
  line L27 (-5.8347, 29.0499) -> (-5.8347, 26.1755)
  line L28 (-5.3247, 29.9999) -> (-5.8347, 29.0499)
  line L29 (-5.8347, 30.9499) -> (-5.3247, 29.9999)
  line L30 (-5.8347, 33.8244) -> (-5.8347, 30.9499)
  arc A27 (-5.8347, 33.8244) -> (-5.9811, 34.178) centre (-6.3347, 33.8244) ccw
  line L31 (-9.9067, 38.1035) -> (-5.9811, 34.178)
  arc A28 (-9.9067, 38.1035) -> (-10.2602, 38.2499) centre (-10.2602, 37.7499) ccw
  line L32 (-12.2428, 38.2499) -> (-10.2602, 38.2499)
  arc A29 (-12.2428, 38.2499) -> (-12.7425, 37.7325) centre (-12.2428, 37.7499) ccw
  line L33 (-12.7425, 34.4374) -> (-12.7425, 37.7325)
  arc A30 (-13.2425, 33.9374) -> (-12.7425, 34.4374) centre (-13.2425, 34.4374) ccw
  line L34 (-14.5, 33.9374) -> (-13.2425, 33.9374)
  arc A31 (-15, 34.4374) -> (-14.5, 33.9374) centre (-14.5, 34.4374) ccw
  line L35 (-15, 42.9999) -> (-15, 34.4374)
  arc A32 (-13, 44.9999) -> (-15, 42.9999) centre (-13, 42.9999) ccw
  line L36 (-4.5625, 44.9999) -> (-13, 44.9999)
  arc A33 (-4.0625, 44.4999) -> (-4.5625, 44.9999) centre (-4.5625, 44.4999) ccw
  line L37 (-4.0625, 43.2424) -> (-4.0625, 44.4999)
  arc A34 (-4.5625, 42.7424) -> (-4.0625, 43.2424) centre (-4.5625, 43.2424) ccw
  line L38 (-7.7325, 42.7424) -> (-4.5625, 42.7424)
  arc A35 (-7.7325, 42.7424) -> (-8.25, 42.2427) centre (-7.75, 42.2427) ccw
  line L39 (-8.25, 40.2601) -> (-8.25, 42.2427)
  arc A36 (-8.25, 40.2601) -> (-8.1035, 39.9066) centre (-7.75, 40.2601) ccw
  line L40 (-4.178, 35.9811) -> (-8.1035, 39.9066)
  arc A37 (-4.178, 35.9811) -> (-3.8245, 35.8346) centre (-3.8245, 36.3346) ccw
  line L41 (-1.0125, 35.8346) -> (-3.8245, 35.8346)
  line L42 (-0.0625, 35.3246) -> (-1.0125, 35.8346)
  line L43 (0.8875, 35.8346) -> (-0.0625, 35.3246)
  line L44 (3.8245, 35.8346) -> (0.8875, 35.8346)
  arc A38 (3.8245, 35.8346) -> (4.178, 35.9811) centre (3.8245, 36.3346) ccw
  line L45 (8.1035, 39.9066) -> (4.178, 35.9811)
  arc A39 (8.1035, 39.9066) -> (8.25, 40.2601) centre (7.75, 40.2601) ccw
  line L46 (8.25, 42.2427) -> (8.25, 40.2601)
  arc A40 (8.25, 42.2427) -> (7.7325, 42.7424) centre (7.75, 42.2427) ccw
  line L47 (4.4375, 42.7424) -> (7.7325, 42.7424)
  arc A41 (3.9375, 43.2424) -> (4.4375, 42.7424) centre (4.4375, 43.2424) ccw
  line L48 (3.9375, 44.4999) -> (3.9375, 43.2424)
  arc A42 (4.4375, 44.9999) -> (3.9375, 44.4999) centre (4.4375, 44.4999) ccw
  line L49 (13, 44.9999) -> (4.4375, 44.9999)
  arc A43 (15, 42.9999) -> (13, 44.9999) centre (13, 42.9999) ccw
  line L50 (15, 34.5624) -> (15, 42.9999)
  arc A44 (14.5, 34.0624) -> (15, 34.5624) centre (14.5, 34.5624) ccw
  line L51 (13.2425, 34.0624) -> (14.5, 34.0624)
  arc A45 (12.7425, 34.5624) -> (13.2425, 34.0624) centre (13.2425, 34.5624) ccw
  line L52 (12.7425, 37.7325) -> (12.7425, 34.5624)
  arc A46 (12.7425, 37.7325) -> (12.2428, 38.2499) centre (12.2428, 37.7499) ccw
  line L53 (10.2602, 38.2499) -> (12.2428, 38.2499)
  arc A47 (10.2602, 38.2499) -> (9.9067, 38.1035) centre (10.2602, 37.7499) ccw
  line L54 (5.9811, 34.178) -> (9.9067, 38.1035)
  arc A48 (5.9811, 34.178) -> (5.8347, 33.8244) centre (6.3347, 33.8244) ccw
  line L55 (5.8347, 30.9499) -> (5.8347, 33.8244)
  line L56 (5.3247, 29.9999) -> (5.8347, 30.9499)
  line L57 (5.8347, 29.0499) -> (5.3247, 29.9999)
  line L58 (5.8347, 26.1755) -> (5.8347, 29.0499)
  arc A49 (5.8347, 26.1755) -> (5.9811, 25.8219) centre (6.3347, 26.1755) ccw
  line L59 (9.9067, 21.8964) -> (5.9811, 25.8219)
  arc A50 (9.9067, 21.8964) -> (10.2602, 21.75) centre (10.2602, 22.25) ccw
  line L60 (12.2428, 21.75) -> (10.2602, 21.75)
  arc A51 (12.2428, 21.75) -> (12.7425, 22.2674) centre (12.2428, 22.25) ccw
  line L61 (12.7425, 25.5624) -> (12.7425, 22.2674)
  arc A52 (13.2425, 26.0624) -> (12.7425, 25.5624) centre (13.2425, 25.5624) ccw
  line L62 (14.5, 26.0624) -> (13.2425, 26.0624)
  arc A53 (15, 25.5624) -> (14.5, 26.0624) centre (14.5, 25.5624) ccw
  line L63 (15, 4.4375) -> (15, 25.5624)
  arc A54 (14.5, 3.9375) -> (15, 4.4375) centre (14.5, 4.4375) ccw
  line L64 (13.2425, 3.9375) -> (14.5, 3.9375)
  arc A55 (12.7425, 4.4375) -> (13.2425, 3.9375) centre (13.2425, 4.4375) ccw
  line L65 (12.7425, 7.7325) -> (12.7425, 4.4375)
  arc A56 (12.7425, 7.7325) -> (12.2428, 8.25) centre (12.2428, 7.75) ccw
  line L66 (10.2602, 8.25) -> (12.2428, 8.25)
  arc A57 (10.2602, 8.25) -> (9.9067, 8.1035) centre (10.2602, 7.75) ccw
  line L67 (5.9811, 4.178) -> (9.9067, 8.1035)
  arc A58 (5.9811, 4.178) -> (5.8347, 3.8245) centre (6.3347, 3.8245) ccw
  line L68 (5.8347, 0.95) -> (5.8347, 3.8245)
  line L69 (5.3247, 0) -> (5.8347, 0.95)
  line L70 (5.8347, -0.95) -> (5.3247, 0)
  line L71 (5.8347, -3.8245) -> (5.8347, -0.95)
  arc A59 (5.8347, -3.8245) -> (5.9811, -4.178) centre (6.3347, -3.8245) ccw
  line L72 (9.9067, -8.1035) -> (5.9811, -4.178)
  arc A60 (9.9067, -8.1035) -> (10.2602, -8.25) centre (10.2602, -7.75) ccw
  line L73 (12.2428, -8.25) -> (10.2602, -8.25)
  arc A61 (12.2428, -8.25) -> (12.7425, -7.7325) centre (12.2428, -7.75) ccw
  line L74 (12.7425, -4.5625) -> (12.7425, -7.7325)
  arc A62 (13.2425, -4.0625) -> (12.7425, -4.5625) centre (13.2425, -4.5625) ccw
  line L75 (14.5, -4.0625) -> (13.2425, -4.0625)
  arc A63 (15, -4.5625) -> (14.5, -4.0625) centre (14.5, -4.5625) ccw
  line L76 (15, -13) -> (15, -4.5625)
  arc A64 (13, -15) -> (15, -13) centre (13, -13) ccw
  line L77 (4.4375, -15) -> (13, -15)
  arc A65 (3.9375, -14.5) -> (4.4375, -15) centre (4.4375, -14.5) ccw
  line L78 (3.9375, -13.2425) -> (3.9375, -14.5)
  arc A66 (4.4375, -12.7425) -> (3.9375, -13.2425) centre (4.4375, -13.2425) ccw
  line L79 (7.7325, -12.7425) -> (4.4375, -12.7425)
  arc A67 (7.7325, -12.7425) -> (8.25, -12.2428) centre (7.75, -12.2428) ccw
  line L80 (8.25, -10.2602) -> (8.25, -12.2428)
  arc A68 (8.25, -10.2602) -> (8.1035, -9.9067) centre (7.75, -10.2602) ccw
  line L81 (4.178, -5.9811) -> (8.1035, -9.9067)
  arc A69 (4.178, -5.9811) -> (3.8245, -5.8347) centre (3.8245, -6.3347) ccw
  line L82 (0.8875, -5.8347) -> (3.8245, -5.8347)
  line L83 (-0.0625, -5.3247) -> (0.8875, -5.8347)
  line L84 (-1.0125, -5.8347) -> (-0.0625, -5.3247)
  line L85 (-3.8245, -5.8347) -> (-1.0125, -5.8347)
  arc A70 (-3.8245, -5.8347) -> (-4.178, -5.9811) centre (-3.8245, -6.3347) ccw
  line L86 (-8.1035, -9.9067) -> (-4.178, -5.9811)
  arc A71 (-8.1035, -9.9067) -> (-8.25, -10.2602) centre (-7.75, -10.2602) ccw
  line L87 (-8.25, -12.2428) -> (-8.25, -10.2602)
  arc A72 (-8.25, -12.2428) -> (-7.7325, -12.7425) centre (-7.75, -12.2428) ccw
  line L88 (-4.5625, -12.7425) -> (-7.7325, -12.7425)
  arc A73 (-4.0625, -13.2425) -> (-4.5625, -12.7425) centre (-4.5625, -13.2425) ccw
  line L89 (-4.0625, -14.5) -> (-4.0625, -13.2425)
  arc A74 (-4.5625, -15) -> (-4.0625, -14.5) centre (-4.5625, -14.5) ccw
  line L90 (-13, -15) -> (-4.5625, -15)
  arc A75 (-15, -13) -> (-13, -15) centre (-13, -13) ccw
  line L91 (-15, -4.4375) -> (-15, -13)
  arc A76 (-14.5, -3.9375) -> (-15, -4.4375) centre (-14.5, -4.4375) ccw
  line L92 (-13.2425, -3.9375) -> (-14.5, -3.9375)
  arc A77 (-12.7425, -4.4375) -> (-13.2425, -3.9375) centre (-13.2425, -4.4375) ccw
  line L93 (-12.7425, -7.7325) -> (-12.7425, -4.4375)
  arc A78 (-12.7425, -7.7325) -> (-12.2428, -8.25) centre (-12.2428, -7.75) ccw
  line L94 (-10.2602, -8.25) -> (-12.2428, -8.25)
  arc A79 (-10.2602, -8.25) -> (-9.9067, -8.1035) centre (-10.2602, -7.75) ccw
  line L95 (-5.9811, -4.178) -> (-9.9067, -8.1035)
  arc A80 (-5.9811, -4.178) -> (-5.8347, -3.8245) centre (-6.3347, -3.8245) ccw
  line L96 (-5.8347, -0.95) -> (-5.8347, -3.8245)
  line L97 (-5.3247, 0) -> (-5.8347, -0.95)
  line L98 (-5.8347, 0.95) -> (-5.3247, 0)
  line L99 (-5.8347, 3.8245) -> (-5.8347, 0.95)
  arc A81 (-5.8347, 3.8245) -> (-5.9811, 4.178) centre (-6.3347, 3.8245) ccw
  line L100 (-9.9067, 8.1035) -> (-5.9811, 4.178)
  arc A82 (-9.9067, 8.1035) -> (-10.2602, 8.25) centre (-10.2602, 7.75) ccw
  line L101 (-12.2428, 8.25) -> (-10.2602, 8.25)
  arc A83 (-12.2428, 8.25) -> (-12.7425, 7.7325) centre (-12.2428, 7.75) ccw
  line L102 (-12.7425, 4.5625) -> (-12.7425, 7.7325)
  arc A84 (-13.2425, 4.0625) -> (-12.7425, 4.5625) centre (-13.2425, 4.5625) ccw
  line L103 (-14.5, 4.0625) -> (-13.2425, 4.0625)
  arc A85 (-15, 4.5625) -> (-14.5, 4.0625) centre (-14.5, 4.5625) ccw
  line L104 (-15, 25.4374) -> (-15, 4.5625)
  arc A86 (-14.5, 25.9374) -> (-15, 25.4374) centre (-14.5, 25.4374) ccw
  line L105 (-13.2425, 25.9374) -> (-14.5, 25.9374)
  arc A87 (-12.7425, 25.4374) -> (-13.2425, 25.9374) centre (-13.2425, 25.4374) ccw
  arc A88 (-9.5, -9.88) -> (-9.88, -9.5) centre (-9.88, -9.88) ccw
  line L106 (-9.88, -9.5) -> (-13.319, -9.5)
  arc A89 (-13.319, -9.5) -> (-13.7, -9.881) centre (-13.319, -9.881) ccw
  line L107 (-13.7, -9.881) -> (-13.7, -12.7)
  arc A90 (-13.7, -12.7) -> (-12.7, -13.7) centre (-12.7, -12.7) ccw
  line L108 (-12.7, -13.7) -> (-9.881, -13.7)
  arc A91 (-9.881, -13.7) -> (-9.5, -13.319) centre (-9.881, -13.319) ccw
  line L109 (-9.5, -13.319) -> (-9.5, -9.88)
  arc A92 (12.8, 19.05) -> (12.3, 19.55) centre (12.3, 19.05) ccw
  line L110 (12.3, 19.55) -> (9.2682, 19.55)
  arc A93 (8.2075, 19.9893) -> (9.2682, 19.55) centre (9.2682, 21.05) ccw
  line L111 (8.2075, 19.9893) -> (4.178, 24.0188)
  arc A94 (4.178, 24.0188) -> (3.8245, 24.1653) centre (3.8245, 23.6653) ccw
  line L112 (3.8245, 24.1653) -> (0.8875, 24.1653)
  line L113 (0.8875, 24.1653) -> (-0.0625, 24.6753)
  line L114 (-0.0625, 24.6753) -> (-1.0125, 24.1653)
  line L115 (-1.0125, 24.1653) -> (-3.8245, 24.1653)
  arc A95 (-3.8245, 24.1653) -> (-4.178, 24.0188) centre (-3.8245, 23.6653) ccw
  line L116 (-4.178, 24.0188) -> (-8.2075, 19.9893)
  arc A96 (-9.2682, 19.55) -> (-8.2075, 19.9893) centre (-9.2682, 21.05) ccw
  line L117 (-9.2682, 19.55) -> (-12.3, 19.55)
  arc A97 (-12.3, 19.55) -> (-12.8, 19.05) centre (-12.3, 19.05) ccw
  line L118 (-12.8, 19.05) -> (-12.8, 10.95)
  arc A98 (-12.8, 10.95) -> (-12.3, 10.45) centre (-12.3, 10.95) ccw
  line L119 (-12.3, 10.45) -> (-9.2682, 10.45)
  arc A99 (-8.2075, 10.0106) -> (-9.2682, 10.45) centre (-9.2682, 8.95) ccw
  line L120 (-8.2075, 10.0106) -> (-4.178, 5.9811)
  arc A100 (-4.178, 5.9811) -> (-3.8245, 5.8347) centre (-3.8245, 6.3347) ccw
  line L121 (-3.8245, 5.8347) -> (-1.0125, 5.8347)
  line L122 (-1.0125, 5.8347) -> (-0.0625, 5.3247)
  line L123 (-0.0625, 5.3247) -> (0.8875, 5.8347)
  line L124 (0.8875, 5.8347) -> (3.8245, 5.8347)
  arc A101 (3.8245, 5.8347) -> (4.178, 5.9811) centre (3.8245, 6.3347) ccw
  line L125 (4.178, 5.9811) -> (8.2075, 10.0106)
  arc A102 (9.2682, 10.45) -> (8.2075, 10.0106) centre (9.2682, 8.95) ccw
  line L126 (9.2682, 10.45) -> (12.3, 10.45)
  arc A103 (12.3, 10.45) -> (12.8, 10.95) centre (12.3, 10.95) ccw
  line L127 (12.8, 10.95) -> (12.8, 19.05)
  arc A104 (-9.88, 39.4999) -> (-9.5, 39.8799) centre (-9.88, 39.8799) ccw
  line L128 (-9.5, 39.8799) -> (-9.5, 43.3189)
  arc A105 (-9.5, 43.3189) -> (-9.881, 43.6999) centre (-9.881, 43.3189) ccw
  line L129 (-9.881, 43.6999) -> (-12.7, 43.6999)
  arc A106 (-12.7, 43.6999) -> (-13.7, 42.6999) centre (-12.7, 42.6999) ccw
  line L130 (-13.7, 42.6999) -> (-13.7, 39.8809)
  arc A107 (-13.7, 39.8809) -> (-13.319, 39.4999) centre (-13.319, 39.8809) ccw
  line L131 (-13.319, 39.4999) -> (-9.88, 39.4999)
  constraints: 1 other
extrude "Body" add sketch "Sketch" along normal up to surface (774.0002 mm away) from surface at 29.9999
sketch "Sketch2" plane through (0, 0, 0) normal (0, 0, 1) x (1, 0, 0)
  line L0 (0, 0) -> (10, 0)
ref_plane "Work Plane3" through (0, 0, 0) normal (0, -1, 0) x (1, 0, 0)
sketch "Sketch3" plane through (0, 0, 0) normal (0, -1, 0) x (1, 0, 0)
  line L0 (-2, 29.9999) -> (12, 29.9999)
  line L1 (-2, 804.0001) -> (12, 804.0001)
  dimension "d7" = 774.0002
  measures "d7" distance between parallel lines of L0 L1
ref_plane "Work Plane6" through (-13, 293, 804.0001) normal (0, 0, 1) x (1, 0, 0)
split "Split3" plane through (-13, 293, 804.0001) removes the side toward (0, 0, 1)
ref_plane "Work Plane7" through (-13, -543, 29.9999) normal (0, 0, -1) x (-1, 0, 0)
split "Split4" plane through (-13, -543, 29.9999) removes the side toward (0, 0, -1)
equation "\"G_OFFSET_START\" = -29.99994"
equation "\"G_OFFSET_END\" = -29.99988"
equation "\"d2\" = -G_OFFSET_START"
equation "\"d3\" = Length + G_OFFSET_END"
equation "\"G_L\" = d7"
equation "\"Length\" = 834"
body "Solid1"
